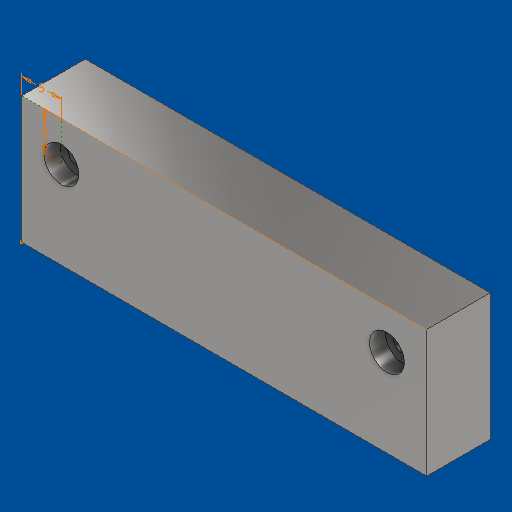
# Autodesk Inventor part: Back Plate
Saved by Autodesk Inventor 2025.1 (Build 291241000, 241)
## iProperties
Created: 2024-12-26
Part Number: Back Plate
Material: Steel, Carbon
Document SubType Name: Modeling
Designer: konch
Density: 7.85 g/cm^3
Appearance: Semi-Polished
Mass: 6.20025 g
Surface Area: 29.2121 cm^2
Volume: 6.20025 cm^3
Description: C55
Author: konch
Autodesk Inventor part; units mm, degrees
ref_plane "YZ Plane" through (0, 0, 0) normal (1, 0, 0) x (0, 1, 0)
ref_plane "XZ Plane" through (0, 0, 0) normal (0, 1, 0) x (-1, 0, 0)
ref_plane "XY Plane" through (0, 0, 0) normal (0, 0, 1) x (1, 0, 0)
sketch "Sketch1" plane through (0, 0, 0) normal (0, 0, 1) x (1, 0, 0)
  line L0 (0, 0) -> (51, 0)
  line L1 (51, 0) -> (51, 16)
  line L2 (51, 16) -> (0, 16)
  line L3 (0, 16) -> (0, 0)
  line L4 (25.5, 0) -> (25.5, 7.5) construction
  line L5 (25.5, 0) -> (25.5, 10.5) construction
  circle A0 centre (25.5, 10.5) radius 4
  dimension "d0" = 51
  dimension "d1" = 16
  dimension "d4" = 10.5
  dimension "d8" = 8
  constraints: 12 end point, 2 perpendicular, 2 vertical, 1 centre point, 1 coincident, 1 horizontal, 1 midpoint, 1 point on line
  measures "d0" distance of L0.start L0.end
  measures "d1" distance of L0.end L1.end
  measures "d4" distance of L4.start L5.end
  measures "d8" diameter of A0
extrude "Extrusion1" add sketch "Sketch1" along normal blind 8 contours L3 L2 L1 L0 | A0
sketch "Sketch2" plane through (0, 0, 0) normal (0, 0, -1) x (-1, 0, 0)
  line L0 (0, 0) -> (-51, 0) construction
  line L1 (-25.5, 0) -> (-25.5, 10.5) construction
  circle A0 centre (-25.5, 10.5) radius 4.75
  line L2 (-25.5, 0) -> (-15.5, 0) construction
  line L3 (-15.5, 0) -> (-15.5, 10.5) construction
  line L4 (-25.5, 0) -> (-35.5, 0) construction
  line L5 (-35.5, 0) -> (-35.5, 10.5) construction
  circle A1 centre (-35.5, 10.5) radius 3
  circle A2 centre (-15.5, 10.5) radius 3
  dimension "d6" = 10.5
  dimension "d7" = 9.5
  dimension "d11" = 10
  dimension "d12" = 10.5
  dimension "d13" = 10
  dimension "d14" = 10.5
  dimension "d15" = 6
  dimension "d16" = 6
  constraints: 10 end point, 3 centre point, 3 coincident, 2 point on line, 1 midpoint, 1 parallel, 1 perpendicular, 1 vertical
  measures "d6" distance of L1.start L1.end
  measures "d7" diameter of A0
  measures "d11" distance of L1.start L2.end
  measures "d12" distance of L2.end L3.end
  measures "d13" distance of L1.start L4.end
  measures "d14" distance of L4.end L5.end
  measures "d15" diameter of A1
  measures "d16" diameter of A2
extrude "Extrusion2" cut sketch "Sketch2" against normal blind 3 contours A0
sketch "Sketch3" plane through (0, 0, 8) normal (0, 0, 1) x (1, 0, 0)
  line L0 (51, 16) -> (0, 16) construction
  line L1 (0, 16) -> (5, 16) construction
  line L2 (5, 16) -> (5, 11) construction
  point P0 (0, 0)
  dimension "d17" = 5
  dimension "d18" = 5
  constraints: 4 end point, 1 point on line, 1 vertical
  measures "d17" distance of L0.end L1.end
  measures "d18" distance of L1.end L2.end
sketch "Sketch4" plane through (0, 0, 8) normal (0, 0, 1) x (1, 0, 0)
  line L0 (51, 16) -> (0, 16) projected
  line L1 (0, 16) -> (0, 11)
  line L2 (0, 16) -> (0, 0) projected
  line L3 (0, 11) -> (5, 11)
  line L4 (51, 16) -> (46, 16)
  line L5 (46, 16) -> (46, 11)
  dimension "d19" = 5
  dimension "d20" = 5
  dimension "d21" = 5
  dimension "d22" = 5
  constraints: 8 end point, 2 coincident, 2 perpendicular, 2 point on line
  measures "d19" distance of L0.end L1.end
  measures "d20" distance of L1.end L3.end
  measures "d21" distance of L0.start L4.end
  measures "d22" distance of L4.end L5.end
hole "Hole1" at (5, 11, 8) at (46, 11, 8) direction (0, 0, -1) diameter 2.4 end through all counterbore diameter 4.4 counterbore depth 2
sketch "Sketch5" plane through (0, 0, 8) normal (0, 0, 1) x (1, 0, 0)
  point P0 (0, 0)
body "Solid1"
